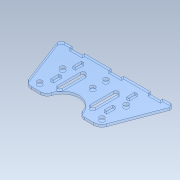
# Autodesk Inventor part: soporte_lateral
Saved by Autodesk Inventor 2022 (Build 260153000, 153)
## iProperties
Created: 2022-11-16
Part Number: soporte_lateral
Material: Generic
Document SubType Name: Modeling
Designer: ferna
Density: 1 g/cm^3
Appearance: Blue - Glazing
Author: ferna
Autodesk Inventor part; units mm, degrees
ref_plane "YZ Plane" through (0, 0, 0) normal (1, 0, 0) x (0, 1, 0)
ref_plane "XZ Plane" through (0, 0, 0) normal (0, 1, 0) x (-1, 0, 0)
ref_plane "XY Plane" through (0, 0, 0) normal (0, 0, 1) x (1, 0, 0)
sketch "Sketch2" plane through (0, 0, 0) normal (0, 1, 0) x (-1, 0, 0)
  line L0 (600, 68.7059) -> (634, 68.7059)
  arc A0 (642, 60.7059) -> (634, 68.7059) centre (634, 60.7059) ccw
  line L1 (642, 60.7059) -> (642, 56.7059)
  arc A1 (634, 48.7059) -> (642, 56.7059) centre (634, 56.7059) ccw
  line L2 (634, 48.7059) -> (632, 48.7059)
  arc A2 (632, 48.7059) -> (624, 40.7059) centre (632, 40.7059) ccw
  line L3 (624, 40.7059) -> (624, 36.7059)
  arc A3 (624, 36.7059) -> (632, 28.7059) centre (632, 36.7059) ccw
  line L4 (632, 28.7059) -> (634, 28.7059)
  arc A4 (642, 20.7059) -> (634, 28.7059) centre (634, 20.7059) ccw
  line L5 (642, 20.7059) -> (642, 16.7059)
  arc A5 (634, 8.7059) -> (642, 16.7059) centre (634, 16.7059) ccw
  line L6 (634, 8.7059) -> (600, 8.7059)
  arc A6 (592, 16.7059) -> (600, 8.7059) centre (600, 16.7059) ccw
  line L7 (592, 16.7059) -> (592, 21.7059)
  line L8 (592, 21.7059) -> (606.1716, 35.8774)
  arc A7 (606.1716, 35.8774) -> (606.1716, 41.5343) centre (603.3431, 38.7059) ccw
  line L9 (606.1716, -97.5343) -> (592, -111.7059)
  line L10 (592, -111.7059) -> (592, -116.7059)
  arc A8 (592, -116.7059) -> (600, -124.7059) centre (600, -116.7059) ccw
  line L11 (600, -124.7059) -> (634, -124.7059)
  arc A9 (634, -124.7059) -> (642, -116.7059) centre (634, -116.7059) ccw
  line L12 (642, -116.7059) -> (642, -112.7059)
  arc A10 (642, -112.7059) -> (634, -104.7059) centre (634, -112.7059) ccw
  line L13 (634, -104.7059) -> (632, -104.7059)
  arc A11 (624, -96.7059) -> (632, -104.7059) centre (632, -96.7059) ccw
  line L14 (624, -96.7059) -> (624, -92.7059)
  arc A12 (632, -84.7059) -> (624, -92.7059) centre (632, -92.7059) ccw
  line L15 (632, -84.7059) -> (634, -84.7059)
  arc A13 (634, -84.7059) -> (642, -76.7059) centre (634, -76.7059) ccw
  line L16 (642, -76.7059) -> (642, -72.7059)
  arc A14 (642, -72.7059) -> (634, -64.7059) centre (634, -72.7059) ccw
  line L17 (634, -64.7059) -> (600, -64.7059)
  arc A15 (600, -64.7059) -> (592, -72.7059) centre (600, -72.7059) ccw
  line L18 (592, -72.7059) -> (592, -77.7059)
  line L19 (592, -77.7059) -> (606.1716, -91.8774)
  arc A16 (606.1716, -97.5343) -> (606.1716, -91.8774) centre (603.3431, -94.7059) ccw
  circle A17 centre (618, -74.7059) radius 3
  circle A18 centre (634, -74.7059) radius 3
  circle A19 centre (634, -114.7059) radius 3
  circle A20 centre (618, -114.7059) radius 3
  circle A21 centre (618, 58.7059) radius 3
  circle A22 centre (634, 58.7059) radius 3
  circle A23 centre (634, 18.7059) radius 3
  circle A24 centre (618, 18.7059) radius 3
  line L20 (606.1716, 41.5343) -> (592, 55.7059)
  line L21 (592, 55.7059) -> (592, 60.7059)
  arc A25 (600, 68.7059) -> (592, 60.7059) centre (600, 60.7059) ccw
  line L22 (329, -137) -> (729, -137)
  line L23 (729, -137) -> (729, 83)
  line L24 (729, 83) -> (329, 83)
  line L25 (329, 83) -> (329, -137)
  line L26 (444, -107.4043) -> (417.5, -107.4043)
  line L27 (417.5, -107.4043) -> (417.5, -104.4043)
  line L28 (417.5, -104.4043) -> (450, -104.4043)
  line L29 (450, -104.4043) -> (450, -107.4043)
  line L30 (450, -107.4043) -> (444, -107.4043)
  line L31 (441, -117.9043) -> (444, -117.9043)
  line L32 (444, -117.9043) -> (444, -110.9043)
  line L33 (444, -110.9043) -> (441, -110.9043)
  line L34 (441, -110.9043) -> (441, -117.9043)
  line L35 (417.5, -121.4043) -> (417.5, -124.4043)
  line L36 (417.5, -124.4043) -> (450, -124.4043)
  line L37 (450, -124.4043) -> (450, -121.4043)
  line L38 (450, -121.4043) -> (417.5, -121.4043)
  line L39 (376.0002, -107.4043) -> (402.5, -107.4043)
  line L40 (402.5, -107.4043) -> (402.5, -104.4043)
  line L41 (402.5, -104.4043) -> (370, -104.4043)
  line L42 (370, -104.4043) -> (370, -107.4043)
  line L43 (370, -107.4043) -> (376.0002, -107.4043)
  line L44 (379.0002, -121.4043) -> (370, -121.4043)
  line L45 (370, -121.4043) -> (370, -124.4043)
  line L46 (370, -124.4043) -> (402.5, -124.4043)
  line L47 (402.5, -124.4043) -> (402.5, -121.4043)
  line L48 (402.5, -121.4043) -> (379.0002, -121.4043)
  line L49 (379.0002, -117.9043) -> (376.0002, -117.9043)
  line L50 (376.0002, -117.9043) -> (376.0002, -110.9043)
  line L51 (376.0002, -110.9043) -> (379.0002, -110.9043)
  line L52 (379.0002, -110.9043) -> (379.0002, -117.9043)
  line L53 (348, -127) -> (472.0002, -127)
  line L54 (472.0002, -127) -> (472.0002, -124.4043)
  line L55 (472.0002, -124.4043) -> (465, -124.4043)
  line L56 (465, -124.4043) -> (465, -121.4043)
  line L57 (465, -121.4043) -> (472.0002, -121.4043)
  line L58 (472.0002, -121.4043) -> (472.0002, -107.4043)
  line L59 (472.0002, -107.4043) -> (465, -107.4043)
  line L60 (465, -107.4043) -> (465, -104.4043)
  line L61 (465, -104.4043) -> (472.0002, -104.4043)
  line L62 (472.0002, -104.4043) -> (472.0002, -101)
  line L63 (472.0002, -101) -> (348, -101)
  line L64 (348, -101) -> (348, -104.4043)
  line L65 (348, -104.4043) -> (355, -104.4043)
  line L66 (355, -104.4043) -> (355, -107.4043)
  line L67 (355, -107.4043) -> (348, -107.4043)
  line L68 (348, -107.4043) -> (348, -121.4043)
  line L69 (348, -121.4043) -> (355, -121.4043)
  line L70 (355, -121.4043) -> (355, -124.4043)
  line L71 (355, -124.4043) -> (348, -124.4043)
  line L72 (348, -124.4043) -> (348, -127)
  circle A26 centre (447.7252, -37.7011) radius 3
  circle A27 centre (372.2748, -37.7011) radius 3
  circle A28 centre (410, -64.4043) radius 3
  circle A29 centre (448.5, -66.4043) radius 3
  circle A30 centre (371.5, -66.4043) radius 3
  circle A31 centre (410, -80.4043) radius 3
  line L73 (379, -84.4043) -> (376, -84.4043)
  line L74 (376, -84.4043) -> (376, -74.4043)
  line L75 (376, -74.4043) -> (379, -74.4043)
  line L76 (379, -74.4043) -> (379, -84.4043)
  line L77 (379, -57.4043) -> (376, -57.4043)
  line L78 (376, -57.4043) -> (376, -47.4043)
  line L79 (376, -47.4043) -> (379, -47.4043)
  line L80 (379, -47.4043) -> (379, -57.4043)
  line L81 (441, -47.4043) -> (441, -57.4043)
  line L82 (441, -57.4043) -> (444, -57.4043)
  line L83 (444, -57.4043) -> (444, -47.4043)
  line L84 (444, -47.4043) -> (441, -47.4043)
  line L85 (441, -74.4043) -> (441, -84.4043)
  line L86 (441, -84.4043) -> (444, -84.4043)
  line L87 (444, -84.4043) -> (444, -74.4043)
  line L88 (444, -74.4043) -> (441, -74.4043)
  line L89 (427, -44.4043) -> (427, -72.4043)
  arc A32 (427, -72.4043) -> (433, -72.4043) centre (430, -72.4043) ccw
  line L90 (433, -72.4043) -> (433, -44.4043)
  arc A33 (433, -44.4043) -> (427, -44.4043) centre (430, -44.4043) ccw
  arc A34 (387, -72.4043) -> (393, -72.4043) centre (390, -72.4043) ccw
  line L91 (393, -72.4043) -> (393, -44.4043)
  arc A35 (393, -44.4043) -> (387, -44.4043) centre (390, -44.4043) ccw
  line L92 (387, -44.4043) -> (387, -72.4043)
  line L93 (372.3983, -27.7019) -> (383.2576, -27.7018)
  arc A36 (390.8984, -33.3311) -> (383.2576, -27.7018) centre (383.2577, -35.7018) ccw
  arc A37 (390.8984, -33.3311) -> (429.1018, -33.3307) centre (410, -27.4043) ccw
  arc A38 (436.7424, -27.7012) -> (429.1018, -33.3307) centre (436.7425, -35.7012) ccw
  line L94 (436.7424, -27.7012) -> (447.7251, -27.7011)
  arc A39 (457.0715, -34.1449) -> (447.7251, -27.7011) centre (447.7252, -37.7011) ccw
  line L95 (457.0715, -34.1449) -> (477.9368, -88.9818)
  arc A40 (474.1982, -94.4043) -> (477.9368, -88.9818) centre (474.1982, -90.4043) ccw
  line L96 (474.1982, -94.4043) -> (465, -94.4043)
  line L97 (465, -94.4043) -> (465, -91.4043)
  line L98 (465, -91.4043) -> (450, -91.4043)
  line L99 (450, -91.4043) -> (450, -94.4043)
  line L100 (450, -94.4043) -> (417.5, -94.4043)
  line L101 (417.5, -94.4043) -> (417.5, -91.4043)
  line L102 (417.5, -91.4043) -> (402.5, -91.4043)
  line L103 (402.5, -91.4043) -> (402.5, -94.4043)
  line L104 (402.5, -94.4043) -> (370, -94.4043)
  line L105 (370, -94.4043) -> (370, -91.4043)
  line L106 (370, -91.4043) -> (355, -91.4043)
  line L107 (355, -91.4043) -> (355, -94.4043)
  line L108 (355, -94.4043) -> (345.8018, -94.4043)
  arc A41 (342.0632, -88.9818) -> (345.8018, -94.4043) centre (345.8018, -90.4043) ccw
  line L109 (342.0632, -88.9818) -> (362.9285, -34.1449)
  arc A42 (372.3983, -27.7019) -> (362.9285, -34.1449) centre (372.2748, -37.7011) ccw
  line L110 (491.3983, -95.7004) -> (502.2576, -95.7005)
  arc A43 (502.2576, -95.7005) -> (509.8984, -90.0712) centre (502.2577, -87.7005) ccw
  arc A44 (548.1018, -90.0716) -> (509.8984, -90.0712) centre (529, -95.998) ccw
  arc A45 (548.1018, -90.0716) -> (555.7424, -95.701) centre (555.7425, -87.701) ccw
  line L111 (555.7424, -95.701) -> (566.7251, -95.7011)
  arc A46 (566.7251, -95.7011) -> (576.0715, -89.2574) centre (566.7252, -85.7011) ccw
  line L112 (576.0715, -89.2574) -> (596.9368, -34.4205)
  arc A47 (596.9368, -34.4205) -> (593.1982, -28.998) centre (593.1982, -32.998) ccw
  line L113 (593.1982, -28.998) -> (584, -28.998)
  line L114 (584, -28.998) -> (584, -31.998)
  line L115 (584, -31.998) -> (569, -31.998)
  line L116 (569, -31.998) -> (569, -28.998)
  line L117 (569, -28.998) -> (536.5, -28.998)
  line L118 (536.5, -28.998) -> (536.5, -31.998)
  line L119 (536.5, -31.998) -> (521.5, -31.998)
  line L120 (521.5, -31.998) -> (521.5, -28.998)
  line L121 (521.5, -28.998) -> (489, -28.998)
  line L122 (489, -28.998) -> (489, -31.998)
  line L123 (489, -31.998) -> (474, -31.998)
  line L124 (474, -31.998) -> (474, -28.998)
  line L125 (474, -28.998) -> (464.8018, -28.998)
  arc A48 (464.8018, -28.998) -> (461.0632, -34.4205) centre (464.8018, -32.998) ccw
  line L126 (461.0632, -34.4205) -> (481.9285, -89.2574)
  arc A49 (481.9285, -89.2574) -> (491.3983, -95.7004) centre (491.2748, -85.7011) ccw
  arc A50 (512, -50.998) -> (506, -50.998) centre (509, -50.998) ccw
  line L127 (512, -50.998) -> (512, -78.998)
  arc A51 (506, -78.998) -> (512, -78.998) centre (509, -78.998) ccw
  line L128 (506, -78.998) -> (506, -50.998)
  line L129 (546, -78.998) -> (546, -50.998)
  arc A52 (552, -50.998) -> (546, -50.998) centre (549, -50.998) ccw
  line L130 (552, -50.998) -> (552, -78.998)
  arc A53 (546, -78.998) -> (552, -78.998) centre (549, -78.998) ccw
  line L131 (560, -48.998) -> (560, -38.998)
  line L132 (560, -38.998) -> (563, -38.998)
  line L133 (563, -38.998) -> (563, -48.998)
  line L134 (563, -48.998) -> (560, -48.998)
  line L135 (560, -75.998) -> (560, -65.998)
  line L136 (560, -65.998) -> (563, -65.998)
  line L137 (563, -65.998) -> (563, -75.998)
  line L138 (563, -75.998) -> (560, -75.998)
  line L139 (498, -65.998) -> (495, -65.998)
  line L140 (495, -65.998) -> (495, -75.998)
  line L141 (495, -75.998) -> (498, -75.998)
  line L142 (498, -75.998) -> (498, -65.998)
  line L143 (498, -38.998) -> (495, -38.998)
  line L144 (495, -38.998) -> (495, -48.998)
  line L145 (495, -48.998) -> (498, -48.998)
  line L146 (498, -48.998) -> (498, -38.998)
  circle A54 centre (529, -42.998) radius 3
  circle A55 centre (490.5, -56.998) radius 3
  circle A56 centre (567.5, -56.998) radius 3
  circle A57 centre (529, -58.998) radius 3
  circle A58 centre (491.2748, -85.7011) radius 3
  circle A59 centre (566.7252, -85.7011) radius 3
  circle A60 centre (462, -114.4043) radius 3
  circle A61 centre (358.0002, -114.4043) radius 3
  line L147 (578, -104.4043) -> (578, -107.4043)
  line L148 (578, -107.4043) -> (585, -107.4043)
  line L149 (585, -107.4043) -> (585, -110.9043)
  line L150 (585, -110.9043) -> (588, -110.9043)
  line L151 (588, -110.9043) -> (588, -117.9043)
  line L152 (588, -117.9043) -> (585, -117.9043)
  line L153 (585, -117.9043) -> (585, -121.4043)
  line L154 (585, -121.4043) -> (578, -121.4043)
  line L155 (578, -121.4043) -> (578, -124.4043)
  line L156 (578, -124.4043) -> (568, -124.4043)
  line L157 (568, -124.4043) -> (568, -121.4043)
  line L158 (568, -121.4043) -> (551, -121.4043)
  line L159 (551, -121.4043) -> (551, -124.4043)
  line L160 (551, -124.4043) -> (541, -124.4043)
  line L161 (541, -124.4043) -> (541, -121.4043)
  line L162 (541, -121.4043) -> (535, -121.4043)
  line L163 (535, -121.4043) -> (535, -107.4043)
  line L164 (535, -107.4043) -> (541, -107.4043)
  line L165 (541, -107.4043) -> (541, -104.4043)
  line L166 (541, -104.4043) -> (551, -104.4043)
  line L167 (551, -104.4043) -> (551, -107.4043)
  line L168 (551, -107.4043) -> (568, -107.4043)
  line L169 (568, -107.4043) -> (568, -104.4043)
  line L170 (568, -104.4043) -> (578, -104.4043)
  line L171 (520, -104.4043) -> (520, -107.4043)
  line L172 (520, -107.4043) -> (527, -107.4043)
  line L173 (527, -107.4043) -> (527, -110.9043)
  line L174 (527, -110.9043) -> (530, -110.9043)
  line L175 (530, -110.9043) -> (530, -117.9043)
  line L176 (530, -117.9043) -> (527, -117.9043)
  line L177 (527, -117.9043) -> (527, -121.4043)
  line L178 (527, -121.4043) -> (520, -121.4043)
  line L179 (520, -121.4043) -> (520, -124.4043)
  line L180 (520, -124.4043) -> (510, -124.4043)
  line L181 (510, -124.4043) -> (510, -121.4043)
  line L182 (510, -121.4043) -> (493, -121.4043)
  line L183 (493, -121.4043) -> (493, -124.4043)
  line L184 (493, -124.4043) -> (483, -124.4043)
  line L185 (483, -124.4043) -> (483, -121.4043)
  line L186 (483, -121.4043) -> (477, -121.4043)
  line L187 (477, -121.4043) -> (477, -107.4043)
  line L188 (477, -107.4043) -> (483, -107.4043)
  line L189 (483, -107.4043) -> (483, -104.4043)
  line L190 (483, -104.4043) -> (493, -104.4043)
  line L191 (493, -104.4043) -> (493, -107.4043)
  line L192 (493, -107.4043) -> (510, -107.4043)
  line L193 (510, -107.4043) -> (510, -104.4043)
  line L194 (510, -104.4043) -> (520, -104.4043)
  line L195 (520, 48.4043) -> (520, 51.4043)
  line L196 (520, 51.4043) -> (527, 51.4043)
  line L197 (527, 51.4043) -> (527, 54.9043)
  line L198 (527, 54.9043) -> (530, 54.9043)
  line L199 (530, 54.9043) -> (530, 61.9043)
  line L200 (530, 61.9043) -> (527, 61.9043)
  line L201 (527, 61.9043) -> (527, 65.4043)
  line L202 (527, 65.4043) -> (520, 65.4043)
  line L203 (520, 65.4043) -> (520, 68.4043)
  line L204 (520, 68.4043) -> (510, 68.4043)
  line L205 (510, 68.4043) -> (510, 65.4043)
  line L206 (510, 65.4043) -> (493, 65.4043)
  line L207 (493, 65.4043) -> (493, 68.4043)
  line L208 (493, 68.4043) -> (483, 68.4043)
  line L209 (483, 68.4043) -> (483, 65.4043)
  line L210 (483, 65.4043) -> (477, 65.4043)
  line L211 (477, 65.4043) -> (477, 51.4043)
  line L212 (477, 51.4043) -> (483, 51.4043)
  line L213 (483, 51.4043) -> (483, 48.4043)
  line L214 (483, 48.4043) -> (493, 48.4043)
  line L215 (493, 48.4043) -> (493, 51.4043)
  line L216 (493, 51.4043) -> (510, 51.4043)
  line L217 (510, 51.4043) -> (510, 48.4043)
  line L218 (510, 48.4043) -> (520, 48.4043)
  line L219 (578, 48.4043) -> (578, 51.4043)
  line L220 (578, 51.4043) -> (585, 51.4043)
  line L221 (585, 51.4043) -> (585, 54.9043)
  line L222 (585, 54.9043) -> (588, 54.9043)
  line L223 (588, 54.9043) -> (588, 61.9043)
  line L224 (588, 61.9043) -> (585, 61.9043)
  line L225 (585, 61.9043) -> (585, 65.4043)
  line L226 (585, 65.4043) -> (578, 65.4043)
  line L227 (578, 65.4043) -> (578, 68.4043)
  line L228 (578, 68.4043) -> (568, 68.4043)
  line L229 (568, 68.4043) -> (568, 65.4043)
  line L230 (568, 65.4043) -> (551, 65.4043)
  line L231 (551, 65.4043) -> (551, 68.4043)
  line L232 (551, 68.4043) -> (541, 68.4043)
  line L233 (541, 68.4043) -> (541, 65.4043)
  line L234 (541, 65.4043) -> (535, 65.4043)
  line L235 (535, 65.4043) -> (535, 51.4043)
  line L236 (535, 51.4043) -> (541, 51.4043)
  line L237 (541, 51.4043) -> (541, 48.4043)
  line L238 (541, 48.4043) -> (551, 48.4043)
  line L239 (551, 48.4043) -> (551, 51.4043)
  line L240 (551, 51.4043) -> (568, 51.4043)
  line L241 (568, 51.4043) -> (568, 48.4043)
  line L242 (568, 48.4043) -> (578, 48.4043)
  circle A62 centre (358.0002, 58.4043) radius 3
  circle A63 centre (462, 58.4043) radius 3
  circle A64 centre (566.7252, 29.7011) radius 3
  circle A65 centre (491.2748, 29.7011) radius 3
  circle A66 centre (529, 2.998) radius 3
  circle A67 centre (567.5, 0.998) radius 3
  circle A68 centre (490.5, 0.998) radius 3
  circle A69 centre (529, -13.002) radius 3
  line L243 (498, -17.002) -> (495, -17.002)
  line L244 (495, -17.002) -> (495, -7.002)
  line L245 (495, -7.002) -> (498, -7.002)
  line L246 (498, -7.002) -> (498, -17.002)
  line L247 (498, 9.998) -> (495, 9.998)
  line L248 (495, 9.998) -> (495, 19.998)
  line L249 (495, 19.998) -> (498, 19.998)
  line L250 (498, 19.998) -> (498, 9.998)
  line L251 (560, 19.998) -> (560, 9.998)
  line L252 (560, 9.998) -> (563, 9.998)
  line L253 (563, 9.998) -> (563, 19.998)
  line L254 (563, 19.998) -> (560, 19.998)
  line L255 (560, -7.002) -> (560, -17.002)
  line L256 (560, -17.002) -> (563, -17.002)
  line L257 (563, -17.002) -> (563, -7.002)
  line L258 (563, -7.002) -> (560, -7.002)
  line L259 (546, 22.998) -> (546, -5.002)
  arc A70 (546, -5.002) -> (552, -5.002) centre (549, -5.002) ccw
  line L260 (552, -5.002) -> (552, 22.998)
  arc A71 (552, 22.998) -> (546, 22.998) centre (549, 22.998) ccw
  arc A72 (506, -5.002) -> (512, -5.002) centre (509, -5.002) ccw
  line L261 (512, -5.002) -> (512, 22.998)
  arc A73 (512, 22.998) -> (506, 22.998) centre (509, 22.998) ccw
  line L262 (506, 22.998) -> (506, -5.002)
  line L263 (491.3983, 39.7004) -> (502.2576, 39.7005)
  arc A74 (509.8984, 34.0712) -> (502.2576, 39.7005) centre (502.2577, 31.7005) ccw
  arc A75 (509.8984, 34.0712) -> (548.1018, 34.0716) centre (529, 39.998) ccw
  arc A76 (555.7424, 39.701) -> (548.1018, 34.0716) centre (555.7425, 31.701) ccw
  line L264 (555.7424, 39.701) -> (566.7251, 39.7011)
  arc A77 (576.0715, 33.2574) -> (566.7251, 39.7011) centre (566.7252, 29.7011) ccw
  line L265 (576.0715, 33.2574) -> (596.9368, -21.5795)
  arc A78 (593.1982, -27.002) -> (596.9368, -21.5795) centre (593.1982, -23.002) ccw
  line L266 (593.1982, -27.002) -> (584, -27.002)
  line L267 (584, -27.002) -> (584, -24.002)
  line L268 (584, -24.002) -> (569, -24.002)
  line L269 (569, -24.002) -> (569, -27.002)
  line L270 (569, -27.002) -> (536.5, -27.002)
  line L271 (536.5, -27.002) -> (536.5, -24.002)
  line L272 (536.5, -24.002) -> (521.5, -24.002)
  line L273 (521.5, -24.002) -> (521.5, -27.002)
  line L274 (521.5, -27.002) -> (489, -27.002)
  line L275 (489, -27.002) -> (489, -24.002)
  line L276 (489, -24.002) -> (474, -24.002)
  line L277 (474, -24.002) -> (474, -27.002)
  line L278 (474, -27.002) -> (464.8018, -27.002)
  arc A79 (461.0632, -21.5795) -> (464.8018, -27.002) centre (464.8018, -23.002) ccw
  line L279 (461.0632, -21.5795) -> (481.9285, 33.2574)
  arc A80 (491.3983, 39.7004) -> (481.9285, 33.2574) centre (491.2748, 29.7011) ccw
  line L280 (372.3983, -28.2981) -> (383.2576, -28.2982)
  arc A81 (383.2576, -28.2982) -> (390.8984, -22.6689) centre (383.2577, -20.2982) ccw
  arc A82 (429.1018, -22.6693) -> (390.8984, -22.6689) centre (410, -28.5957) ccw
  arc A83 (429.1018, -22.6693) -> (436.7424, -28.2988) centre (436.7425, -20.2988) ccw
  line L281 (436.7424, -28.2988) -> (447.7251, -28.2989)
  arc A84 (447.7251, -28.2989) -> (457.0715, -21.8551) centre (447.7252, -18.2989) ccw
  line L282 (457.0715, -21.8551) -> (477.9368, 32.9818)
  arc A85 (477.9368, 32.9818) -> (474.1982, 38.4043) centre (474.1982, 34.4043) ccw
  line L283 (474.1982, 38.4043) -> (465, 38.4043)
  line L284 (465, 38.4043) -> (465, 35.4043)
  line L285 (465, 35.4043) -> (450, 35.4043)
  line L286 (450, 35.4043) -> (450, 38.4043)
  line L287 (450, 38.4043) -> (417.5, 38.4043)
  line L288 (417.5, 38.4043) -> (417.5, 35.4043)
  line L289 (417.5, 35.4043) -> (402.5, 35.4043)
  line L290 (402.5, 35.4043) -> (402.5, 38.4043)
  line L291 (402.5, 38.4043) -> (370, 38.4043)
  line L292 (370, 38.4043) -> (370, 35.4043)
  line L293 (370, 35.4043) -> (355, 35.4043)
  line L294 (355, 35.4043) -> (355, 38.4043)
  line L295 (355, 38.4043) -> (345.8018, 38.4043)
  arc A86 (345.8018, 38.4043) -> (342.0632, 32.9818) centre (345.8018, 34.4043) ccw
  line L296 (342.0632, 32.9818) -> (362.9285, -21.8551)
  arc A87 (362.9285, -21.8551) -> (372.3983, -28.2981) centre (372.2748, -18.2989) ccw
  arc A88 (393, 16.4043) -> (387, 16.4043) centre (390, 16.4043) ccw
  line L297 (393, 16.4043) -> (393, -11.5957)
  arc A89 (387, -11.5957) -> (393, -11.5957) centre (390, -11.5957) ccw
  line L298 (387, -11.5957) -> (387, 16.4043)
  line L299 (427, -11.5957) -> (427, 16.4043)
  arc A90 (433, 16.4043) -> (427, 16.4043) centre (430, 16.4043) ccw
  line L300 (433, 16.4043) -> (433, -11.5957)
  arc A91 (427, -11.5957) -> (433, -11.5957) centre (430, -11.5957) ccw
  line L301 (441, 18.4043) -> (441, 28.4043)
  line L302 (441, 28.4043) -> (444, 28.4043)
  line L303 (444, 28.4043) -> (444, 18.4043)
  line L304 (444, 18.4043) -> (441, 18.4043)
  line L305 (441, -8.5957) -> (441, 1.4043)
  line L306 (441, 1.4043) -> (444, 1.4043)
  line L307 (444, 1.4043) -> (444, -8.5957)
  line L308 (444, -8.5957) -> (441, -8.5957)
  line L309 (379, 1.4043) -> (376, 1.4043)
  line L310 (376, 1.4043) -> (376, -8.5957)
  line L311 (376, -8.5957) -> (379, -8.5957)
  line L312 (379, -8.5957) -> (379, 1.4043)
  line L313 (379, 28.4043) -> (376, 28.4043)
  line L314 (376, 28.4043) -> (376, 18.4043)
  line L315 (376, 18.4043) -> (379, 18.4043)
  line L316 (379, 18.4043) -> (379, 28.4043)
  circle A92 centre (410, 24.4043) radius 3
  circle A93 centre (371.5, 10.4043) radius 3
  circle A94 centre (448.5, 10.4043) radius 3
  circle A95 centre (410, 8.4043) radius 3
  circle A96 centre (372.2748, -18.2989) radius 3
  circle A97 centre (447.7252, -18.2989) radius 3
  line L317 (348, 71) -> (472.0002, 71)
  line L318 (472.0002, 71) -> (472.0002, 68.4043)
  line L319 (472.0002, 68.4043) -> (465, 68.4043)
  line L320 (465, 68.4043) -> (465, 65.4043)
  line L321 (465, 65.4043) -> (472.0002, 65.4043)
  line L322 (472.0002, 65.4043) -> (472.0002, 51.4043)
  line L323 (472.0002, 51.4043) -> (465, 51.4043)
  line L324 (465, 51.4043) -> (465, 48.4043)
  line L325 (465, 48.4043) -> (472.0002, 48.4043)
  line L326 (472.0002, 48.4043) -> (472.0002, 45)
  line L327 (472.0002, 45) -> (348, 45)
  line L328 (348, 45) -> (348, 48.4043)
  line L329 (348, 48.4043) -> (355, 48.4043)
  line L330 (355, 48.4043) -> (355, 51.4043)
  line L331 (355, 51.4043) -> (348, 51.4043)
  line L332 (348, 51.4043) -> (348, 65.4043)
  line L333 (348, 65.4043) -> (355, 65.4043)
  line L334 (355, 65.4043) -> (355, 68.4043)
  line L335 (355, 68.4043) -> (348, 68.4043)
  line L336 (348, 68.4043) -> (348, 71)
  line L337 (379.0002, 61.9043) -> (376.0002, 61.9043)
  line L338 (376.0002, 61.9043) -> (376.0002, 54.9043)
  line L339 (376.0002, 54.9043) -> (379.0002, 54.9043)
  line L340 (379.0002, 54.9043) -> (379.0002, 61.9043)
  line L341 (379.0002, 65.4043) -> (370, 65.4043)
  line L342 (370, 65.4043) -> (370, 68.4043)
  line L343 (370, 68.4043) -> (402.5, 68.4043)
  line L344 (402.5, 68.4043) -> (402.5, 65.4043)
  line L345 (402.5, 65.4043) -> (379.0002, 65.4043)
  line L346 (376.0002, 51.4043) -> (402.5, 51.4043)
  line L347 (402.5, 51.4043) -> (402.5, 48.4043)
  line L348 (402.5, 48.4043) -> (370, 48.4043)
  line L349 (370, 48.4043) -> (370, 51.4043)
  line L350 (370, 51.4043) -> (376.0002, 51.4043)
  line L351 (417.5, 65.4043) -> (417.5, 68.4043)
  line L352 (417.5, 68.4043) -> (450, 68.4043)
  line L353 (450, 68.4043) -> (450, 65.4043)
  line L354 (450, 65.4043) -> (417.5, 65.4043)
  line L355 (441, 61.9043) -> (444, 61.9043)
  line L356 (444, 61.9043) -> (444, 54.9043)
  line L357 (444, 54.9043) -> (441, 54.9043)
  line L358 (441, 54.9043) -> (441, 61.9043)
  line L359 (444, 51.4043) -> (417.5, 51.4043)
  line L360 (417.5, 51.4043) -> (417.5, 48.4043)
  line L361 (417.5, 48.4043) -> (450, 48.4043)
  line L362 (450, 48.4043) -> (450, 51.4043)
  line L363 (450, 51.4043) -> (444, 51.4043)
  line L364 (672, -101.5) -> (672, -103)
  line L365 (672, -103) -> (695, -103)
  line L366 (695, -103) -> (695, -107.1363)
  arc A98 (692.2891, -110.9229) -> (695, -107.1363) centre (691, -107.1363) ccw
  line L367 (692.2891, -110.9229) -> (650.6445, -125.0997)
  arc A99 (648, -123.2064) -> (650.6445, -125.0997) centre (650, -123.2064) ccw
  line L368 (648, -123.2064) -> (648, -115)
  line L369 (648, -115) -> (649, -115)
  arc A100 (649, -115) -> (651, -113) centre (649, -113) ccw
  line L370 (651, -113) -> (651, -90)
  arc A101 (651, -90) -> (649, -88) centre (649, -90) ccw
  line L371 (649, -88) -> (648, -88)
  line L372 (648, -88) -> (648, -79.7936)
  arc A102 (650.6445, -77.9003) -> (648, -79.7936) centre (650, -79.7936) ccw
  line L373 (650.6445, -77.9003) -> (692.2891, -92.0771)
  arc A103 (695, -95.8637) -> (692.2891, -92.0771) centre (691, -95.8637) ccw
  line L374 (695, -95.8637) -> (695, -100)
  line L375 (695, -100) -> (672, -100)
  line L376 (672, -100) -> (672, -101.5)
  line L377 (671, 47.5) -> (671, 46)
  line L378 (671, 46) -> (694, 46)
  line L379 (694, 46) -> (694, 41.8637)
  arc A104 (691.2891, 38.0771) -> (694, 41.8637) centre (690, 41.8637) ccw
  line L380 (691.2891, 38.0771) -> (649.6445, 23.9003)
  arc A105 (647, 25.7936) -> (649.6445, 23.9003) centre (649, 25.7936) ccw
  line L381 (647, 25.7936) -> (647, 34)
  line L382 (647, 34) -> (648, 34)
  arc A106 (648, 34) -> (650, 36) centre (648, 36) ccw
  line L383 (650, 36) -> (650, 59)
  arc A107 (650, 59) -> (648, 61) centre (648, 59) ccw
  line L384 (648, 61) -> (647, 61)
  line L385 (647, 61) -> (647, 69.2064)
  arc A108 (649.6445, 71.0997) -> (647, 69.2064) centre (649, 69.2064) ccw
  line L386 (649.6445, 71.0997) -> (691.2891, 56.9229)
  arc A109 (694, 53.1363) -> (691.2891, 56.9229) centre (690, 53.1363) ccw
  line L387 (694, 53.1363) -> (694, 49)
  line L388 (694, 49) -> (671, 49)
  line L389 (671, 49) -> (671, 47.5)
  line L390 (692.5332, 13) -> (713, 13)
  line L391 (713, 13) -> (713, 28)
  line L392 (713, 28) -> (716, 28)
  line L393 (716, 28) -> (716, 37.1982)
  arc A110 (716, 37.1982) -> (710.5775, 40.9368) centre (712, 37.1982) ccw
  line L394 (710.5775, 40.9368) -> (655.7406, 20.0715)
  arc A111 (655.7406, 20.0715) -> (649.7575, 13.7252) centre (659.2969, 10.7252) ccw
  line L395 (649.7575, 13.7252) -> (659.2969, 13.7252)
  arc A112 (659.2969, 7.7252) -> (659.2969, 13.7252) centre (659.2969, 10.7252) ccw
  line L396 (659.2969, 7.7252) -> (649.2969, 7.7252)
  line L397 (649.2969, 7.7252) -> (649.2963, 1.7997)
  arc A113 (677.6446, -24) -> (649.2963, 1.7997) centre (649, -27) ccw
  line L398 (677.6446, -24) -> (686, -24)
  arc A114 (686.0452, -29.9997) -> (686, -24) centre (686, -27) ccw
  line L399 (686.0452, -29.9997) -> (677.6446, -29.9997)
  arc A115 (649.2975, -55.7997) -> (677.6446, -29.9997) centre (649, -27) ccw
  line L400 (649.2975, -55.7997) -> (649.2976, -61.7252)
  line L401 (649.2976, -61.7252) -> (659.2969, -61.7252)
  arc A116 (659.2969, -67.7252) -> (659.2969, -61.7252) centre (659.2969, -64.7252) ccw
  line L402 (659.2969, -67.7252) -> (649.7575, -67.7252)
  arc A117 (649.7575, -67.7252) -> (655.7406, -74.0715) centre (659.2969, -64.7252) ccw
  line L403 (655.7406, -74.0715) -> (710.5775, -94.9368)
  arc A118 (710.5775, -94.9368) -> (716, -91.1982) centre (712, -91.1982) ccw
  line L404 (716, -91.1982) -> (716, -82)
  line L405 (716, -82) -> (713, -82)
  line L406 (713, -82) -> (713, -67)
  line L407 (713, -67) -> (692.5332, -67)
  line L408 (692.5332, -67) -> (692.5332, -64)
  line L409 (692.5332, -64) -> (716, -64)
  line L410 (716, -64) -> (716, -34.5)
  line L411 (716, -34.5) -> (713, -34.5)
  line L412 (713, -34.5) -> (713, -19.5)
  line L413 (713, -19.5) -> (716, -19.5)
  line L414 (716, -19.5) -> (716, 10)
  line L415 (716, 10) -> (692.5332, 10)
  line L416 (692.5332, 10) -> (692.5332, 13)
  point P0 (0, 0)
  point P1 (461.0632, -21.5795)
  point P2 (593.1982, -27.002)
  point P3 (576.0715, 33.2574)
  point P4 (548.1018, 34.0716)
  point P5 (509.8984, 34.0712)
  point P6 (481.9285, 33.2574)
  point P7 (506, -5.002)
  point P8 (506, 22.998)
  point P9 (512, -5.002)
  point P10 (552, -5.002)
  constraints: 834 end point, 166 point on circle, 119 centre point
extrude "Extrusion2" add sketch "Sketch2" along normal blind 3 contours L263 A74 A75 A76 L264 A77 L265 A78 L266 L267 L268 L269 L270 L271 L272 L273 L274 L275 L276 L277 L278 A79 L279 A80
body "Solid2"
